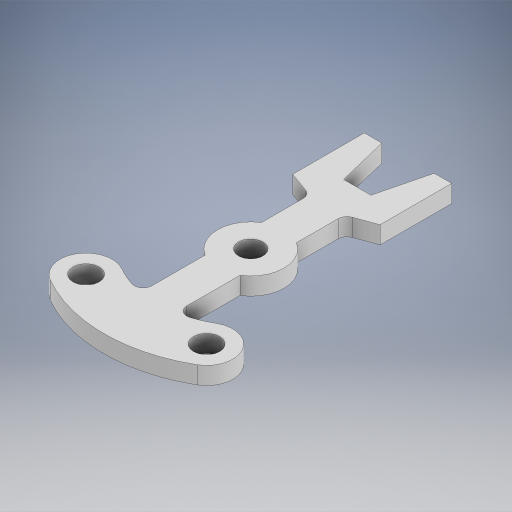
# Autodesk Inventor part: 1.2 pt 1
Saved by Autodesk Inventor 2024 (Build 280153000, 153)
## iProperties
Created: 2024-01-18
Part Number: 1.2 pt 1
Material: Generic
Document SubType Name: Modeling
Designer: Alex
Density: 1 g/cm^3
Appearance: Default
Author: Alex
Autodesk Inventor part; units mm, degrees
ref_plane "YZ Plane" through (0, 0, 0) normal (1, 0, 0) x (0, 1, 0)
ref_plane "XZ Plane" through (0, 0, 0) normal (0, 1, 0) x (-1, 0, 0)
ref_plane "XY Plane" through (0, 0, 0) normal (0, 0, 1) x (1, 0, 0)
sketch "Sketch1" plane through (0, 0, 0) normal (0, 1, 0) x (-1, 0, 0)
  circle A0 centre (0, 0) radius 7
  circle A1 centre (0, 0) radius 69 construction
  line L0 (0, 0) -> (-34.5, 59.7558) construction
  line L1 (0, 0) -> (69, 0) construction
  circle A2 centre (-34.5, 59.7558) radius 7.5
  arc A3 (-42, 72.7461) -> (-27, 46.7654) centre (-34.5, 59.7558) ccw
  circle A4 centre (0, 0) radius 84 construction
  line L2 (0, -84) -> (0, 84) construction
  circle A5 centre (34.5, 59.7558) radius 7.5
  arc A6 (27, 46.7654) -> (42, 72.7461) centre (34.5, 59.7558) ccw
  arc A7 (42, 72.7461) -> (-42, 72.7461) centre (0, 0) ccw
  arc A8 (-10, -53.066) -> (27, 46.7654) centre (0, 0) ccw construction
  line L3 (10, -83.4026) -> (-10, -83.4026) construction
  line L4 (-10, -83.4026) -> (-10, -40.0394) construction
  line L5 (-10, 83.4026) -> (10, 83.4026) construction
  line L6 (10, 83.4026) -> (10, 46.6476) construction
  line L7 (10, -83.4026) -> (-10, 83.4026) construction
  line L8 (-10, -83.4026) -> (10, 83.4026) construction
  arc A9 (-10, 46.6476) -> (-16.5306, 51.4076) centre (-15, 46.6476) ccw
  arc A10 (16.5306, 51.4076) -> (10, 46.6476) centre (15, 46.6476) ccw
  arc A11 (-27, 46.7654) -> (-10, -53.066) centre (0, 0) ccw construction
  line L9 (-10, 46.6476) -> (-10, 83.4026) construction
  line L10 (10, 46.6476) -> (10, 16.1555)
  line L11 (10, 16.1555) -> (10, -16.1555) construction
  line L12 (10, -16.1555) -> (10, -83.4026) construction
  line L13 (-10, 16.1555) -> (-10, 46.6476)
  arc A12 (-10, 16.1555) -> (-10, -16.1555) centre (0, 0) ccw
  arc A13 (-16.5306, 51.4076) -> (-27, 46.7654) centre (0, 0) ccw
  arc A14 (27, 46.7654) -> (16.5306, 51.4076) centre (0, 0) ccw
  line L14 (-19, 0) -> (19, 0) construction
  line L15 (-10, 0) -> (10, 0) construction
  line L16 (10, 0) -> (10, -90) construction
  line L17 (10, -90) -> (-10, -90) construction
  line L18 (-10, -90) -> (-10, 0) construction
  line L19 (-10, 0) -> (10, 0) construction
  line L20 (10, 0) -> (10, -61) construction
  line L21 (10, -61) -> (0, -61) construction
  line L22 (-10, -61) -> (-10, -40.0394) construction
  line L23 (0, -90) -> (-25, -90) construction
  line L24 (0, -90) -> (-15, -90) construction
  line L25 (0, -90) -> (15, -90) construction
  line L26 (-15, -90) -> (15, -90) construction
  line L27 (-15, -90) -> (-7.7695, -61)
  line L28 (-15, -90) -> (14.8878, -90) construction
  line L29 (-25, -90) -> (-25, -49)
  line L30 (-25, -90) -> (16, -90) construction
  line L31 (-25, -49) -> (-13.2899, -44.7379)
  line L32 (-25, -49) -> (-9.0373, -49) construction
  arc A15 (-13.2899, -44.7379) -> (-10, -40.0394) centre (-15, -40.0394) ccw
  line L33 (-10, -40.0394) -> (-10, -16.1555) construction
  line L34 (-13.2899, -44.7379) -> (-10, -43.5404) construction
  line L35 (-10, -40.0394) -> (-10, -16.1555)
  line L36 (-25, -90) -> (-15, -90)
  line L37 (-7.7695, -61) -> (-10, -61) construction
  line L38 (0, -61) -> (-7.7695, -61)
  line L39 (-10, -16.1555) -> (-10, 0) construction
  line L40 (-10, -16.1555) -> (-10, 16.1555) construction
  line L41 (0, -90) -> (25, -90) construction
  line L42 (15, -90) -> (7.7695, -61)
  line L43 (25, -90) -> (25, -49)
  line L44 (25, -90) -> (-16, -90) construction
  line L45 (25, -49) -> (13.2899, -44.7379)
  arc A16 (10, -40.0394) -> (13.2899, -44.7379) centre (15, -40.0394) ccw
  line L46 (10, -40.0394) -> (10, -16.1555) construction
  line L47 (10, -40.0394) -> (10, -16.1555)
  line L48 (0, -61) -> (7.7695, -61)
  arc A17 (10, -16.1555) -> (10, 16.1555) centre (0, 0) ccw
  line L49 (25, -90) -> (15, -90)
  dimension "d2" = 138
  dimension "d0" = 14
  dimension "d3" = 120
  dimension "d4" = 15
  dimension "d5" = 30
  dimension "d6" = 20
  dimension "d7" = 10
  dimension "d9" = 20
  dimension "d10" = 90
  dimension "d11" = 20
  dimension "d12" = 61
  dimension "d13" = 25
  dimension "d16" = 15
  dimension "d17" = 180
  dimension "d20" = 76
  dimension "d21" = 90
  dimension "d22" = 5
  dimension "d23" = 41
  dimension "d24" = 90
  dimension "d25" = 20
  dimension "d26" = 10
  dimension "d27" = 19
  dimension "d28" = 19
  constraints: 100 end point, 33 point on circle, 29 parallel, 17 centre point, 14 tangent, 10 horizontal, 10 symmetric about line, 8 point on line, 7 coincident, 7 perpendicular, 4 equal length, 4 midpoint, 2 vertical, 7 other
  measures "d0" diameter of A0
  measures "d3" angle of L1 L0
  measures "d4" diameter of A2
  measures "d5" diameter of A3
  measures "d6" distance of L5.start L5.end
  measures "d7" diameter of A9
  measures "d9" distance of L16.end L17.end
  measures "d10" distance of L15.end L16.end
  measures "d11" distance of L20.end L22.start
  measures "d12" distance of L19.end L20.end
  measures "d13" distance of L23.start L23.end
  measures "d16" distance of L23.start L24.end
  measures "d17" angle of L24 L25
  measures "d20" angle of L28 L27
  measures "d21" angle of L24 L11
  measures "d22" distance from line of L26.end L11
  measures "d23" distance of L23.end L29.end
  measures "d24" angle of L30 L29
  measures "d25" angle of L32 L31
  measures "d26" diameter of A15
  measures "d27" radius of A17
  measures "d28" radius of A12
extrude "Extrusion1" add sketch "Sketch1" along normal blind 10
body "Solid1"
